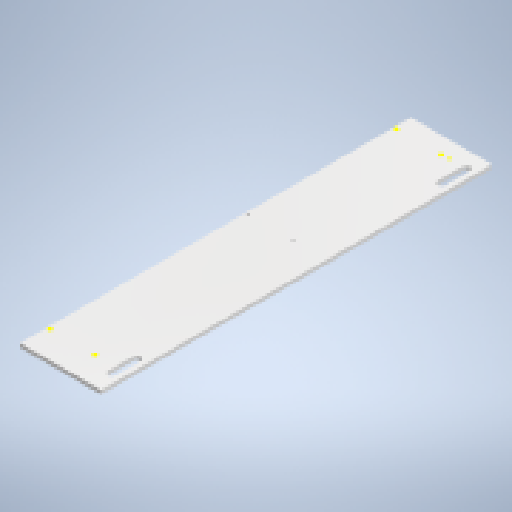
# Autodesk Inventor part: Plexi_Teileband
Saved by Autodesk Inventor 2025 (Build 290162000, 162)
## iProperties
Created: 2025-08-17
Part Number: Plexi_Teileband
Material: Generic
Document SubType Name: Modeling
Designer: peter
Density: 1 g/cm^3
Appearance: Default
Author: peter
Autodesk Inventor part; units mm, degrees
ref_plane "YZ Plane" through (0, 0, 0) normal (1, 0, 0) x (0, 1, 0)
ref_plane "XZ Plane" through (0, 0, 0) normal (0, 1, 0) x (-1, 0, 0)
ref_plane "XY Plane" through (0, 0, 0) normal (0, 0, 1) x (1, 0, 0)
sketch "Sketch2" plane through (0, 0, 0) normal (0, 0, 1) x (1, 0, 0)
  circle A0 centre (-16.5, -300) radius 3 projected
  circle A1 centre (-106.5, -300) radius 3 projected
  line L0 (-4.5, -755) -> (-112.5, -755) projected
  line L1 (-4.5, -585) -> (-4.5, -755) projected
  line L2 (-4.5, -585) -> (-6, -585) projected
  line L3 (-6, -585) -> (-6, -582) projected
  line L4 (-6, -582) -> (1.5, -582) projected
  line L5 (1.5, -38) -> (1.5, -582) projected
  line L6 (1.5, -38) -> (-6, -38) projected
  line L7 (-6, -38) -> (-6, -35) projected
  line L8 (-6, -35) -> (-4.5, -35) projected
  line L9 (-4.5, 35) -> (-4.5, -35) projected
  line L10 (-112.5, 35) -> (-4.5, 35) projected
  line L11 (-112.5, -755) -> (47.5, -755)
  line L12 (47.5, -755) -> (47.5, 35)
  line L13 (47.5, 35) -> (-112.5, 35)
  line L14 (-112.5, 35) -> (-112.5, -755)
  line L15 (-112.5, -755) -> (-112.5, 35) projected
  circle A2 centre (-16.5, -700) radius 3 projected
  circle A3 centre (-106.5, 0) radius 3 projected
  circle A4 centre (-106.5, -700) radius 3 projected
  circle A5 centre (-16.5, 0) radius 3 projected
  point P0 (0, 0)
  dimension "d3" = 160
  constraints: 8 end point, 2 parallel, 1 horizontal, 1 horizontal alignment, 1 perpendicular
  measures "d3" distance of L13.end L12.end
extrude "Extrusion1" add sketch "Sketch2" along normal blind 8 contours L0 L14 L10 L9 L8 L7 L6 L5 L4 L3 L2 L1 | L1 L2 L3 L4 L5 L6 L7 L8 L9 L13 L12 L11 | A2 | A3 | A4 | A5
sketch "Sketch3" plane through (0, 0, 8) normal (0, 0, 1) x (1, 0, 0)
  line L0 (33, -749.6938) -> (33, 23.1387) construction
  line L1 (47.5, -755) -> (47.5, 35) construction
  line L2 (33, -714.5754) -> (33, -663.8389) construction
  line L3 (40.7469, -714.5754) -> (40.7469, -663.8389)
  line L4 (25.2531, -663.8389) -> (25.2531, -714.5754)
  arc A0 (25.2531, -714.5754) -> (40.7469, -714.5754) centre (33, -714.5754) ccw
  arc A1 (40.7469, -663.8389) -> (25.2531, -663.8389) centre (33, -663.8389) ccw
  line L5 (33, 1.707) -> (33, -48.3122) construction
  line L6 (40.7469, 1.707) -> (40.7469, -48.3122)
  line L7 (25.2531, -48.3122) -> (25.2531, 1.707)
  arc A2 (40.7469, 1.707) -> (25.2531, 1.707) centre (33, 1.707) ccw
  arc A3 (25.2531, -48.3122) -> (40.7469, -48.3122) centre (33, -48.3122) ccw
  point P0 (0, 0)
  point P1 (33, -689.2072)
  point P2 (33, -23.3026)
  dimension "d4" = 14.5
  constraints: 18 end point, 8 point on circle, 8 tangent, 4 centre point, 4 point on line, 3 parallel, 2 midpoint
  measures "d4" distance between parallel lines of L1 L0
extrude "Extrusion2" cut sketch "Sketch3" against normal through all
thicken "Thicken1" operation add thickness 4 both sides no extend neighbours no toward (1, 0, 0) faces at (47.5, -491.6667, 2.6667)
fillet "Fillet1" radius 2 2 edges at (51.5, 35, 4) (51.5, -755, 4)
sketch "Sketch4" plane through (0, 0, 8) normal (0, 0, 1) x (1, 0, 0)
  circle A0 centre (-16.5, 0) radius 3 projected
  circle A1 centre (-106.5, 0) radius 3 projected
  circle A2 centre (-16.5, -700) radius 3 projected
  circle A3 centre (-106.5, -700) radius 3 projected
  point P0 (0, 0)
extrude "Extrusion3" cut sketch "Sketch4" against normal blind 10
body "Solid1"
